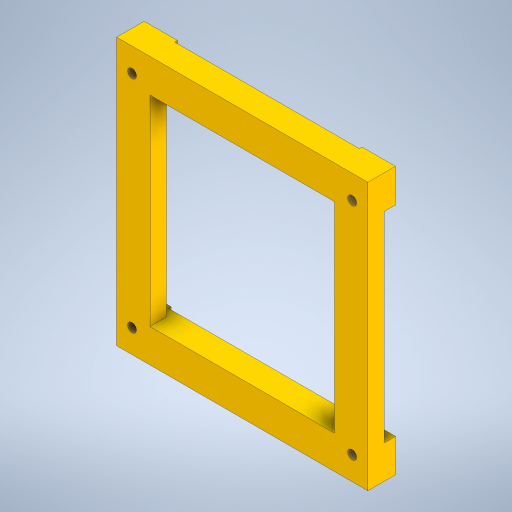
# Autodesk Inventor part: ThomasBracket v2
Saved by Autodesk Inventor 2023 (Build 270158000, 158)
## iProperties
Created: 2023-04-13
Part Number: ThomasBracket v2
Material: Generic
Document SubType Name: Sheet Metal
Designer: User
Density: 1 g/cm^3
Sheet Metal Rule: Default
Appearance: Default
Author: User
Autodesk Inventor part; units mm, degrees
ref_plane "YZ Plane" through (0, 0, 0) normal (1, 0, 0) x (0, 1, 0)
ref_plane "XZ Plane" through (0, 0, 0) normal (0, 1, 0) x (-1, 0, 0)
ref_plane "XY Plane" through (0, 0, 0) normal (0, 0, 1) x (1, 0, 0)
sketch "Sketch1" plane through (0, 0, 0) normal (0, 0, 1) x (1, 0, 0)
  line L0 (-10.2061, 4.9951) -> (79.9639, 4.9951)
  line L1 (79.9639, 4.9951) -> (79.9639, -90.8899)
  line L2 (79.9639, -90.8899) -> (-10.2061, -90.8899)
  line L3 (-10.2061, -90.8899) -> (-10.2061, 4.9951)
  line L4 (67.9639, -78.8899) -> (1.7939, -78.8899)
  line L5 (67.9639, -78.8899) -> (67.9639, -7.0049)
  line L6 (67.9639, -7.0049) -> (1.7939, -7.0049)
  line L7 (1.7939, -7.0049) -> (1.7939, -78.8899)
  point P0 (0, 0)
  dimension "d0" = 90.17
  dimension "d1" = 95.885
  constraints: 16 end point, 2 parallel, 1 horizontal, 1 perpendicular
  measures "d0" distance of L1.end L2.end
  measures "d1" distance of L0.end L1.end
extrude "Extrusion1" add sketch "Sketch1" along normal blind 9.906
sketch "Sketch2" plane through (0, 0, 9.906) normal (0, 0, 1) x (1, 0, 0)
  circle A0 centre (-4.6211, -82.4449) radius 1.6
  circle A1 centre (74.3789, -82.4449) radius 1.6
  circle A2 centre (-4.6211, -3.4499) radius 1.6
  circle A3 centre (74.3789, -3.4499) radius 1.6
  line L0 (79.9639, 4.9951) -> (-10.2061, 4.9951) projected
  line L1 (-10.2061, -90.8899) -> (79.9639, -90.8899) projected
  line L2 (79.9639, -90.8899) -> (79.9639, 4.9951) projected
  line L3 (-10.2061, 4.9951) -> (-10.2061, -90.8899) projected
  point P0 (0, 0)
  dimension "d18" = 3.2
  dimension "d19" = 3.2
  dimension "d20" = 3.2
  dimension "d21" = 3.2
  dimension "d22" = 8.445
  dimension "d23" = 8.445
  dimension "d24" = 8.445
  dimension "d25" = 8.445
  dimension "d26" = 5.585
  dimension "d27" = 5.585
  dimension "d28" = 5.585
  dimension "d29" = 5.585
  constraints: 4 centre point
  measures "d18" diameter of A0
  measures "d19" diameter of A1
  measures "d20" diameter of A2
  measures "d21" diameter of A3
  measures "d22" distance from line of L0 A3.centre
  measures "d23" distance from line of L0 A2.centre
  measures "d24" distance from line of L1 A0.centre
  measures "d25" distance from line of L1 A1.centre
  measures "d26" distance from line of L2 A1.centre
  measures "d27" distance from line of L3 A0.centre
  measures "d28" distance from line of L2 A3.centre
  measures "d29" distance from line of L3 A2.centre
extrude "Extrusion2" cut sketch "Sketch2" against normal blind 3.302 contours A0 | A1 | A2 | A3
thread "Thread1" size "6-32 UNC" class "2B" standard "ANSI Unified Screw Threads" full length
thread "Thread2" size "6-32 UNC" class "2B" standard "ANSI Unified Screw Threads" full length
thread "Thread3" size "6-32 UNC" class "2B" standard "ANSI Unified Screw Threads" full length
thread "Thread4" size "6-32 UNC" class "2B" standard "ANSI Unified Screw Threads" full length
sketch "Sketch3" plane through (0, 0, 0) normal (0, 0, -1) x (-1, 0, 0)
  circle A0 centre (-71.0739, -0.0849) radius 1.524
  circle A1 centre (5.1261, -85.8099) radius 1.524
  circle A2 centre (-74.8839, -85.8099) radius 1.524
  circle A3 centre (2.5861, -0.0849) radius 1.524
  line L0 (-79.9639, 4.9951) -> (10.2061, 4.9951) projected
  line L1 (-79.9639, -90.8899) -> (-79.9639, 4.9951) projected
  line L2 (10.2061, -90.8899) -> (-79.9639, -90.8899) projected
  line L3 (10.2061, 4.9951) -> (10.2061, -90.8899) projected
  point P0 (0, 0)
  dimension "d40" = 3.048
  dimension "d41" = 3.048
  dimension "d42" = 3.048
  dimension "d43" = 3.048
  dimension "d45" = 8.89
  dimension "d46" = 90.805
  dimension "d47" = 5.08
  dimension "d48" = 5.08
  dimension "d50" = 85.09
  dimension "d51" = 5.08
  dimension "d52" = 82.55
  dimension "d53" = 90.805
  constraints: 4 centre point
  measures "d40" diameter of A0
  measures "d41" diameter of A1
  measures "d42" diameter of A2
  measures "d43" diameter of A3
  measures "d45" distance from line of L1 A0.centre
  measures "d46" distance from line of L2 A0.centre
  measures "d47" distance from line of L2 A2.centre
  measures "d48" distance from line of L1 A2.centre
  measures "d50" distance from line of L1 A1.centre
  measures "d51" distance from line of L2 A1.centre
  measures "d52" distance from line of L1 A3.centre
  measures "d53" distance from line of L2 A3.centre
extrude "Extrusion3" cut sketch "Sketch3" against normal blind 3.302 contours A0 | A1 | A2 | A3
sketch "Sketch4" plane through (0, 0, 0) normal (0, 0, -1) x (-1, 0, 0)
  line L0 (-1.7939, -7.0049) -> (-67.9639, -7.0049) projected
  line L1 (-1.7939, -7.0049) -> (10.2061, -7.0049)
  line L2 (10.2061, 4.9951) -> (10.2061, -90.8899) projected
  line L3 (-1.7939, -78.8899) -> (10.2061, -78.8899)
  line L4 (-67.9639, -78.8899) -> (-1.7939, -78.8899) projected
  line L5 (10.2061, -78.8899) -> (-67.9639, -78.8899)
  line L6 (-67.9639, -78.8899) -> (-79.9639, -78.8899)
  line L7 (-79.9639, -90.8899) -> (-79.9639, 4.9951) projected
  line L8 (-67.9639, -7.0049) -> (-79.9639, -7.0049)
  line L9 (-67.9639, -7.0049) -> (-67.9639, -78.8899) projected
  line L10 (-67.9639, -7.8922) -> (-67.9639, -78.8899)
  line L11 (-67.9639, -78.8899) -> (-79.9639, -78.8899)
  line L12 (-1.7939, -7.0049) -> (-67.9639, -7.0049) projected
  line L13 (-79.9639, -7.0049) -> (-1.7939, -7.0049)
  line L14 (-1.7939, -78.8899) -> (-1.7939, -7.0049) projected
  line L15 (-1.7939, -7.0049) -> (-1.7939, -78.8899)
  line L16 (-1.7939, -78.8899) -> (10.2061, -78.8899)
  point P0 (0, 0)
  constraints: 20 end point, 6 point on line, 3 collinear, 3 perpendicular, 2 horizontal
extrude "Extrusion4" cut sketch "Sketch4" against normal blind 4 contours L1 L2 L3 L14 | L9 L6 L7 L8
sketch "Sketch5" plane through (0, 0, 0) normal (0, 0, -1) x (-1, 0, 0)
  line L0 (-79.9639, 4.9951) -> (10.2061, 4.9951) projected
  circle A0 centre (-71.0739, -0.0849) radius 1.524 projected
  circle A1 centre (2.5861, -0.0849) radius 1.524 projected
  line L1 (-1.7939, -7.0049) -> (-67.9639, -7.0049) projected
  line L2 (-1.7939, -7.0049) -> (-1.7939, 4.9951)
  line L3 (-67.9639, -7.0049) -> (-67.9639, 4.9951)
  line L4 (-67.9639, -7.0049) -> (-67.9639, -78.8899) projected
  line L5 (-67.9639, -78.8899) -> (-67.9639, -90.8899)
  line L6 (10.2061, -90.8899) -> (-79.9639, -90.8899) projected
  line L7 (-67.9639, -78.8899) -> (-1.7939, -78.8899) projected
  line L8 (-1.7939, -78.8899) -> (-1.7939, -90.8899)
  point P0 (0, 0)
  constraints: 8 end point, 5 point on line, 1 perpendicular, 1 vertical
extrude "Extrusion5" cut sketch "Sketch5" against normal blind 1 contours L7 L8 L6 L5 | L0 L2 L1 L3
sketch "Sketch6" plane through (0, 0, 0) normal (0, 0, -1) x (-1, 0, 0)
  line L0 (0.5761, -90.8899) -> (0.5761, -83.261)
  circle A0 centre (-74.8839, -85.8099) radius 1.524 projected
  circle A1 centre (5.1261, -85.8099) radius 1.524 projected
  line L1 (0.5761, -83.261) -> (0.5761, -78.8899)
  line L2 (10.2061, -78.8899) -> (-1.7939, -78.8899) projected
  line L3 (-70.3339, -87.0755) -> (-70.3339, -90.8899)
  line L4 (-70.3339, -87.0755) -> (-70.3339, -78.8899)
  line L5 (-67.9639, -78.8899) -> (-79.9639, -78.8899) projected
  line L6 (10.2061, -90.8899) -> (-79.9639, -90.8899) projected
  line L7 (-67.9639, -90.8899) -> (-67.9639, -78.8899)
  line L8 (-70.3339, -78.8899) -> (-70.3339, -90.8899)
  line L9 (-1.7939, -90.8899) -> (0.5761, -90.8899)
  line L10 (-67.9639, -78.8899) -> (-1.7939, -78.8899) projected
  line L11 (0.5761, -78.8899) -> (-1.7939, -78.8899)
  line L12 (-1.7939, -78.8899) -> (-1.7939, -90.8899) projected
  line L13 (-1.7939, -78.8899) -> (-1.7939, -90.8899)
  point P0 (0, 0)
  dimension "d63" = 4.55
  constraints: 18 end point, 5 point on line, 2 collinear, 2 perpendicular, 1 horizontal, 1 vertical
  measures "d63" distance from line of L0 A1.centre
extrude "Extrusion6" cut sketch "Sketch6" against normal blind 1 contours L6 L12 L2 L1 L0 | L6 L3 L4 L5 L7
thread "Thread5" size "5-40 UNC" class "2B" standard "ANSI Unified Screw Threads" full length
thread "Thread6" size "5-40 UNC" class "2B" standard "ANSI Unified Screw Threads" full length
thread "Thread7" size "5-40 UNC" class "2B" standard "ANSI Unified Screw Threads" full length
thread "Thread8" size "5-40 UNC" class "2B" standard "ANSI Unified Screw Threads" full length
equation "\"BendRadius\" = Thickness"
equation "\"BendReliefWidth\" = Thickness"
equation "\"BendReliefDepth\" = 0.5 * Thickness"
equation "\"CornerReliefSize\" = 4 * Thickness"
equation "\"MinimumRemnant\" = 2 * Thickness"
equation "\"TransitionRadius\" = BendRadius"
equation "\"JacobiRadiusSize\" = BendRadius"
equation "\"GapSize\" = Thickness"
equation "\"Thickness\" = 3.048"
body "Solid1"
